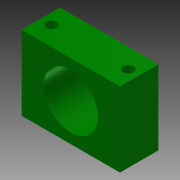
# Autodesk Inventor part: 2.5 CIM mount
Saved by Autodesk Inventor 2013 (Build 170138000, 138)
## iProperties
Created: 2013-01-18
Part Number: 2.5 CIM mount
Material: Polypropylene
Document SubType Name: Modeling
Designer: Naphat
Density: 0.899 g/cm^3
Mass: 258.943 g
Surface Area: 469.405 cm^2
Volume: 288.035 cm^3
Author: Naphat
Autodesk Inventor part; units mm, degrees
ref_plane "YZ Plane" through (0, 0, 0) normal (1, 0, 0) x (0, 1, 0)
ref_plane "XZ Plane" through (0, 0, 0) normal (0, 1, 0) x (-1, 0, 0)
ref_plane "XY Plane" through (0, 0, 0) normal (0, 0, 1) x (1, 0, 0)
sketch "Sketch20" plane through (0, 0, 0) normal (0, 1, 0) x (-1, 0, 0)
  line L0 (57.5, -22.5) -> (-57.5, -22.5)
  line L1 (-57.5, -22.5) -> (-57.5, 22.5)
  line L2 (-57.5, 22.5) -> (57.5, 22.5)
  line L3 (57.5, 22.5) -> (57.5, -22.5)
  circle A0 centre (45, 0) radius 6
  circle A1 centre (-45, 0) radius 6
  point P0 (0, 0)
  dimension "d92" = 115
  dimension "d93" = 45
  dimension "d94" = 57.5
  dimension "d95" = 22.5
  dimension "d97" = 45
  dimension "d98" = 90
  dimension "d99" = 12
  dimension "d100" = 12
  constraints: 8 end point, 2 centre point, 2 horizontal alignment, 2 parallel, 1 horizontal, 1 perpendicular
  measures "d92" distance between parallel lines of L3 L1
  measures "d93" distance between parallel lines of L0 L2
  measures "d94" distance from line of point (0, 0) L3
  measures "d95" distance from line of point (0, 0) L2
  measures "d97" distance of A1.centre point (0, 0)
  measures "d98" distance of A1.centre A0.centre
  measures "d99" diameter of A0
  measures "d100" diameter of A1
extrude "Extrusion17" add sketch "Sketch20" along normal blind 87
sketch "Sketch21" plane through (57.5, 0, -22.5) normal (0, 0, -1) x (-1, 0, 0)
  line L0 (115, 0) -> (115, 87) projected
  line L1 (0, 87) -> (115, 87) projected
  line L2 (0, 0) -> (0, 87) projected
  line L3 (57.5, 0) -> (57.5, 87) construction
  line L4 (115, 43.5) -> (0, 43.5) construction
  circle A0 centre (57.5, 43.5) radius 31.75
  dimension "d103" = 63.5
  constraints: 4 end point, 4 midpoint, 1 centre point
  measures "d103" diameter of A0
hole "Hole1" at (0, 43.5, -22.5) direction (0, 0, 1) diameter 63.5 end through all
equation "\"d94\" = 0.5 * d92"
equation "\"d95\" = 0.5 * d93"
equation "\"d97\" = 0.5 * d98"
equation "\"d100\" = d99"
body "Solid3"
